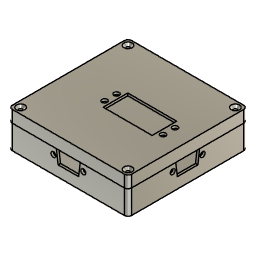
TRARM02_Base (Autodesk Fusion 360 design; units mm, degrees)
Autodesk Fusion 360 part; units mm, degrees
sketch "스케치1" plane through (0, 0, 0) normal (0, 0, 1) x (1, 0, 0) in component "TRARM02_Base_Bottom_100x100x20 v1"
  line L0 (0, 0) -> (100, 0)
  line L1 (100, 0) -> (100, 100)
  line L2 (100, 100) -> (0, 100)
  line L3 (0, 100) -> (0, 0)
  dimension "d25" = 100
  dimension "d26" = 100
  constraint horizontal L0
  constraint vertical L1
  constraint horizontal L2
  constraint vertical L3
  constraint coincident L0.start L3.end
  measures "d25" distance of L0.start L0.end
  measures "d26" distance of L0.start L2.end
extrude "돌출4" add sketch "스케치1" along normal blind 2 makes body 1 in component "TRARM02_Base_Bottom_100x100x20 v1"
sketch "스케치7" plane through (0, 0, 2) normal (0, 0, 1) x (-1, 0, 0) in component "TRARM02_Base_Bottom_100x100x20 v1"
  line L0 (0, -100) -> (-100, -100)
  line L1 (-100, -100) -> (-100, 0)
  line L2 (-100, 0) -> (0, 0)
  line L3 (0, 0) -> (0, -100)
  line L4 (-10, -98) -> (-90, -98)
  line L5 (-98, -90) -> (-98, -10)
  line L6 (-90, -2) -> (-10, -2)
  line L7 (-2, -10) -> (-2, -90)
  line L8 (-2, -90) -> (-10, -90)
  line L9 (-10, -90) -> (-10, -98)
  line L10 (-90, -98) -> (-90, -90)
  line L11 (-90, -90) -> (-98, -90)
  line L12 (-2, -10) -> (-10, -10)
  line L13 (-10, -10) -> (-10, -2)
  line L14 (-90, -2) -> (-90, -10)
  line L15 (-90, -10) -> (-98, -10)
  point P0 (0, -100)
  point P1 (-100, 0)
  dimension "d46" = 2
  dimension "d47" = 2
  dimension "d49" = 2
  dimension "d50" = 2
  dimension "d85" = 10
  dimension "d86" = 10
  dimension "d91" = 10
  dimension "d92" = 10
  constraint horizontal L0
  constraint vertical L1
  constraint horizontal L2
  constraint vertical L3
  constraint coincident P1 L1.end
  constraint coincident P0 L0.start
  constraint horizontal L4
  constraint vertical L5
  constraint horizontal L6
  constraint vertical L7
  constraint perpendicular L7 L8
  constraint perpendicular L4 L9
  constraint perpendicular L4 L10
  constraint perpendicular L5 L11
  constraint perpendicular L7 L12
  constraint perpendicular L6 L13
  constraint perpendicular L6 L14
  constraint perpendicular L5 L15
  constraint equal L9 L10
  constraint equal L8 L11
  constraint equal L13 L14
  constraint equal L12 L15
  measures "d46" distance of L3 L7
  measures "d47" distance of L0 L4
  measures "d49" distance of L1 L5
  measures "d50" distance of L2 L6
  measures "d85" distance of P0 L9
  measures "d86" distance of P0 L8
  measures "d91" distance of P1 L14
  measures "d92" distance of P1 L15
extrude "돌출7" add sketch "스케치7" along normal blind 18 bodies 1 in component "TRARM02_Base_Bottom_100x100x20 v1"
fillet "모깎기1" radius 3 4 edges at (100, 0, 10) (0, 0, 10) (100, 100, 10) (0, 100, 10) on bodies 1 in component "TRARM02_Base_Bottom_100x100x20 v1"
fillet "모깎기1" radius 3 4 edges at (10, 90, 11) (10, 10, 11) (90, 10, 11) (90, 90, 11) on bodies 1 in component "TRARM02_Base_Bottom_100x100x20 v1"
sketch "스케치9" plane through (0, 0, 0) normal (0, -1, 0) x (1, 0, 0) in component "TRARM02_Base_Bottom_100x100x20 v1"
  line L0 (41.4, 9) -> (40, 20)
  line L1 (90, 20) -> (10, 20)
  line L2 (41.4, 9) -> (58.6, 9)
  line L3 (58.6, 9) -> (60, 20)
  line L4 (40, 20) -> (60, 20)
  circle A0 centre (62.5, 14.5) radius 2.1
  circle A1 centre (37.5, 14.5) radius 2.1
  point P0 (50, 20)
  point P1 (10, 20)
  point P2 (90, 20)
  dimension "d72" = 17.2
  dimension "d73" = 50
  dimension "d74" = 20
  dimension "d75" = 11
  dimension "d76" = 4.2
  dimension "d77" = 4.2
  dimension "d78" = 25
  dimension "d81" = 5.5
  dimension "d82" = 12.5
  constraint coincident L1 P0
  constraint coincident L3.end L1
  constraint coincident L1 L0.end
  constraint midpoint P0 L4
  constraint equal L0 L3
  constraint horizontal A0.centre A1.centre
  measures "d72" distance of L0.start L2.end
  measures "d73" horizontal distance of origin P0
  measures "d74" distance of L3.end L0.end
  measures "d75" distance of L2 L4
  measures "d76" diameter of A0
  measures "d77" diameter of A1
  measures "d78" distance of A0.centre A1.centre
  measures "d81" distance of L2 A1.centre
  measures "d82" horizontal distance of P0 A1.centre
extrude "돌출9" cut sketch "스케치9" against normal blind 100 bodies 1 in component "TRARM02_Base_Bottom_100x100x20 v1"
sketch "스케치11" plane through (0, 0, 20) normal (0, 0, 1) x (-1, 0, 0) in component "TRARM02_Base_Bottom_100x100x20 v1"
  circle A0 centre (-5, -95) radius 1.45
  circle A1 centre (-95, -95) radius 1.45
  circle A2 centre (-95, -5) radius 1.45
  circle A3 centre (-5, -5) radius 1.45
  line L0 (0, -97) -> (0, -3)
  line L1 (-3, 0) -> (-40, 0)
  line L2 (-60, 0) -> (-97, 0)
  line L3 (-100, -3) -> (-100, -97)
  line L4 (-97, -100) -> (-60, -100)
  line L5 (-40, -100) -> (-3, -100)
  line L6 (-97, -100) -> (-60, -100)
  dimension "d93" = 2.9
  dimension "d103" = 5
  dimension "d108" = 2.9
  dimension "d109" = 90
  dimension "d110" = 90
  constraint horizontal A0.centre A1.centre
  constraint equal A2 A3
  constraint vertical A0.centre A3.centre
  constraint horizontal A2.centre A3.centre
  constraint vertical A1.centre A2.centre
  constraint equal A0 A1
  measures "d93" diameter of A3
  measures "d103" distance of A0.centre L0
  measures "d108" diameter of A0
  measures "d109" distance of A0.centre A1.centre
  measures "d110" distance of A0.centre A3.centre
extrude "돌출10" cut sketch "스케치11" against normal blind 20 bodies 1 in component "TRARM02_Base_Bottom_100x100x20 v1"
sketch "스케치12" plane through (0, 0, 0) normal (-1, 0, 0) x (0, -1, 0) in component "TRARM02_Base_Bottom_100x100x20 v1"
  line L0 (-58.6, 9) -> (-41.4, 9)
  circle A0 centre (-62.5, 14.5) radius 2.1
  line L1 (-58.6, 9) -> (-60, 20)
  line L2 (-60, 20) -> (-40, 20)
  line L3 (-41.4, 9) -> (-40, 20)
  circle A1 centre (-37.5, 14.5) radius 2.1
  line L4 (-97, 20) -> (-3, 20)
  point P0 (-64, 20)
  point P1 (-100, 0)
  point P2 (-50, 20)
  point P3 (-90, 20)
  dimension "d115" = 17.2
  dimension "d117" = 20
  dimension "d118" = 11
  dimension "d119" = 4.2
  dimension "d120" = 4.2
  dimension "d121" = 25
  dimension "d122" = 5.5
  dimension "d123" = 12.5
  dimension "d124" = 50
  constraint midpoint P2 L2
  constraint equal L1 L3
  constraint horizontal A1.centre A0.centre
  constraint parallel L2 L4
  constraint coincident P2 L4
  measures "d115" distance of L0.start L0.end
  measures "d117" distance of L2.end L1.end
  measures "d118" distance of L0 L2
  measures "d119" diameter of A1
  measures "d120" diameter of A0
  measures "d121" distance of A1.centre A0.centre
  measures "d122" distance of A0.centre L0
  measures "d123" horizontal distance of A0.centre P2
  measures "d124" horizontal distance of origin P2
extrude "돌출11" cut sketch "스케치12" against normal blind 100 bodies 1 in component "TRARM02_Base_Bottom_100x100x20 v1"
sketch "스케치1 (2)" plane through (0, 0, 0) normal (0, 0, 1) x (1, 0, 0) in component "TRARM02_Base_Top_100x100x10 v1"
  line L0 (0, 0) -> (100, 0)
  line L1 (100, 0) -> (100, 100)
  line L2 (100, 100) -> (0, 100)
  line L3 (0, 100) -> (0, 0)
  dimension "d1" = 100
  dimension "d2" = 100
  constraint horizontal L0
  constraint vertical L1
  constraint horizontal L2
  constraint vertical L3
  constraint coincident L0.start L3.end
  measures "d1" distance of L0.start L0.end
  measures "d2" distance of L0.start L2.end
extrude "돌출1" add sketch "스케치1 (2)" along normal blind 2 separate body makes body 2 in component "TRARM02_Base_Top_100x100x10 v1"
sketch "스케치2" plane through (0, 0, 2) normal (0, 0, 1) x (-1, 0, 0) in component "TRARM02_Base_Top_100x100x10 v1"
  line L0 (0, -100) -> (-100, -100)
  line L1 (-100, -100) -> (-100, 0)
  line L2 (-100, 0) -> (0, 0)
  line L3 (0, 0) -> (0, -100)
  line L4 (-10, -98) -> (-90, -98)
  line L5 (-98, -90) -> (-98, -10)
  line L6 (-90, -2) -> (-10, -2)
  line L7 (-2, -10) -> (-2, -90)
  line L8 (-2, -90) -> (-10, -90)
  line L9 (-10, -90) -> (-10, -98)
  line L10 (-90, -98) -> (-90, -90)
  line L11 (-90, -90) -> (-98, -90)
  line L12 (-98, -10) -> (-90, -10)
  line L13 (-90, -10) -> (-90, -2)
  line L14 (-10, -2) -> (-10, -10)
  line L15 (-10, -10) -> (-2, -10)
  point P0 (0, -100)
  point P1 (-100, 0)
  dimension "d5" = 2
  dimension "d6" = 2
  dimension "d7" = 8
  dimension "d8" = 8
  dimension "d9" = 2
  dimension "d10" = 2
  dimension "d11" = 8
  dimension "d12" = 8
  constraint horizontal L0
  constraint vertical L1
  constraint horizontal L2
  constraint vertical L3
  constraint coincident P1 L1.end
  constraint coincident P0 L0.start
  constraint horizontal L4
  constraint vertical L5
  constraint horizontal L6
  constraint vertical L7
  constraint perpendicular L7 L8
  constraint perpendicular L4 L9
  constraint perpendicular L4 L10
  constraint perpendicular L5 L11
  constraint perpendicular L5 L12
  constraint perpendicular L6 L13
  constraint perpendicular L6 L14
  constraint perpendicular L7 L15
  constraint equal L11 L12
  constraint equal L9 L14
  constraint equal L13 L14
  constraint equal L8 L11
  measures "d5" distance of L3 L7
  measures "d6" distance of L2 L6
  measures "d7" distance of L14.end L7.start
  measures "d8" distance of L6.end L14.end
  measures "d9" distance of L1 L5
  measures "d10" distance of L0 L4
  measures "d11" distance of L10.end L5.start
  measures "d12" distance of L4.end L10.end
extrude "돌출2" add sketch "스케치2" along normal blind 8 bodies 2 in component "TRARM02_Base_Top_100x100x10 v1"
sketch "스케치3" plane through (0, 0, 10) normal (0, 0, 1) x (-1, 0, 0) in component "TRARM02_Base_Top_100x100x10 v1"
  circle A0 centre (-5, -95) radius 1.5
  circle A1 centre (-95, -95) radius 1.5
  circle A2 centre (-95, -5) radius 1.5
  circle A3 centre (-5, -5) radius 1.5
  dimension "d15" = 3
  dimension "d16" = 5
  dimension "d17" = 5
  dimension "d18" = 90
  dimension "d19" = 90
  constraint equal A2 A3
  constraint equal A0 A1
  constraint equal A1 A2
  constraint horizontal A2.centre A3.centre
  constraint vertical A1.centre A2.centre
  constraint vertical A0.centre A3.centre
  constraint horizontal A0.centre A1.centre
  measures "d15" diameter of A0
  measures "d16" horizontal distance of origin A3.centre
  measures "d17" vertical distance of origin A3.centre
  measures "d18" distance of A2.centre A3.centre
  measures "d19" distance of A0.centre A3.centre
extrude "돌출3" cut sketch "스케치3" against normal blind 10 bodies 2 in component "TRARM02_Base_Top_100x100x10 v1"
fillet "필렛1" radius 3 4 edges at (0, 0, 5) (100, 0, 5) (100, 100, 5) (0, 100, 5) on bodies 2 in component "TRARM02_Base_Top_100x100x10 v1"
fillet "필렛1" radius 3 4 edges at (10, 90, 6) (10, 10, 6) (90, 90, 6) (90, 10, 6) on bodies 2 in component "TRARM02_Base_Top_100x100x10 v1"
chamfer "챔퍼1" distance 2 angle 45 4 edges at (6.3985, 95.5424, 0) (6.3985, 5.5424, 0) (96.3985, 5.5424, 0) (96.3985, 95.5424, 0) on bodies 2 in component "TRARM02_Base_Top_100x100x10 v1"
sketch "스케치4" plane through (0, 0, 2) normal (0, 0, 1) x (-1, 0, 0) in component "TRARM02_Base_Top_100x100x10 v1"
  line L0 (-39.5, -60.3) -> (-80.5, -60.3)
  line L1 (-80.5, -60.3) -> (-80.5, -39.7)
  line L2 (-80.5, -39.7) -> (-39.5, -39.7)
  line L3 (-39.5, -39.7) -> (-39.5, -60.3)
  circle A0 centre (-35.5, -55.1) radius 2.25
  circle A1 centre (-35.5, -45.1) radius 2.25
  circle A2 centre (-84.5, -55.1) radius 2.25
  circle A3 centre (-84.5, -45.1) radius 2.25
  point P0 (-3, -100)
  dimension "d27_1" = 20.6
  dimension "d28_1" = 41
  dimension "d29" = 39.5
  dimension "d33" = 10
  dimension "d34" = 49
  dimension "d35" = 4.5
  dimension "d37" = 5.4
  dimension "d41" = 39.7
  dimension "d43" = 4
  constraint horizontal L0
  constraint vertical L1
  constraint horizontal L2
  constraint vertical L3
  constraint equal A2 A3
  constraint equal A0 A2
  constraint equal A0 A1
  constraint horizontal A0.centre A2.centre
  constraint vertical A0.centre A1.centre
  constraint horizontal A1.centre A3.centre
  constraint vertical A2.centre A3.centre
  measures "d27_1" distance of L0.end L1.end
  measures "d28_1" distance of L1.end L2.end
  measures "d29" horizontal distance of origin L2.end
  measures "d33" distance of A0.centre A1.centre
  measures "d34" distance of A0.centre A2.centre
  measures "d35" diameter of A2
  measures "d37" vertical distance of L2.end A1.centre
  measures "d41" vertical distance of origin L2.end
  measures "d43" horizontal distance of L2.end A1.centre
extrude "돌출4'" cut sketch "스케치4" against normal blind 2 bodies 2 in component "TRARM02_Base_Top_100x100x10 v1"
component "TRARM02_Base_Bottom_100x100x20 v1" placed x (1, 0, 0) y (0, 1, 0) z (0, 0, 1) at (-50, -50, 0)
component "TRARM02_Base_Top_100x100x10 v1" placed x (1, 0, 0) y (0, -1, 0) z (0, 0, -1) at (-50, 50, 30)
